Autodesk Fusion 360 part; units mm, degrees
note: some values were not read from the file. Chosen so that the rebuilt part matches the saved one: which bodies a step acts on.
(part 3 of 3)
  constraint symmetric L133.end L135 A142.end
  constraint symmetric A140 L135 A143
  constraint symmetric A141 L135 A142
  measures "d112" diameter of A138
  measures "d113" diameter of A139
  measures "d114" distance of A140.centre P0
  measures "d115" diameter of A140
extrude "Extrude8" cut sketch "Sketch8" against normal blind 5 contours A138 | A139 | L132 A140 L133 A141 | A142 L136 L137 A143 bodies 2
named bodies: "base"
